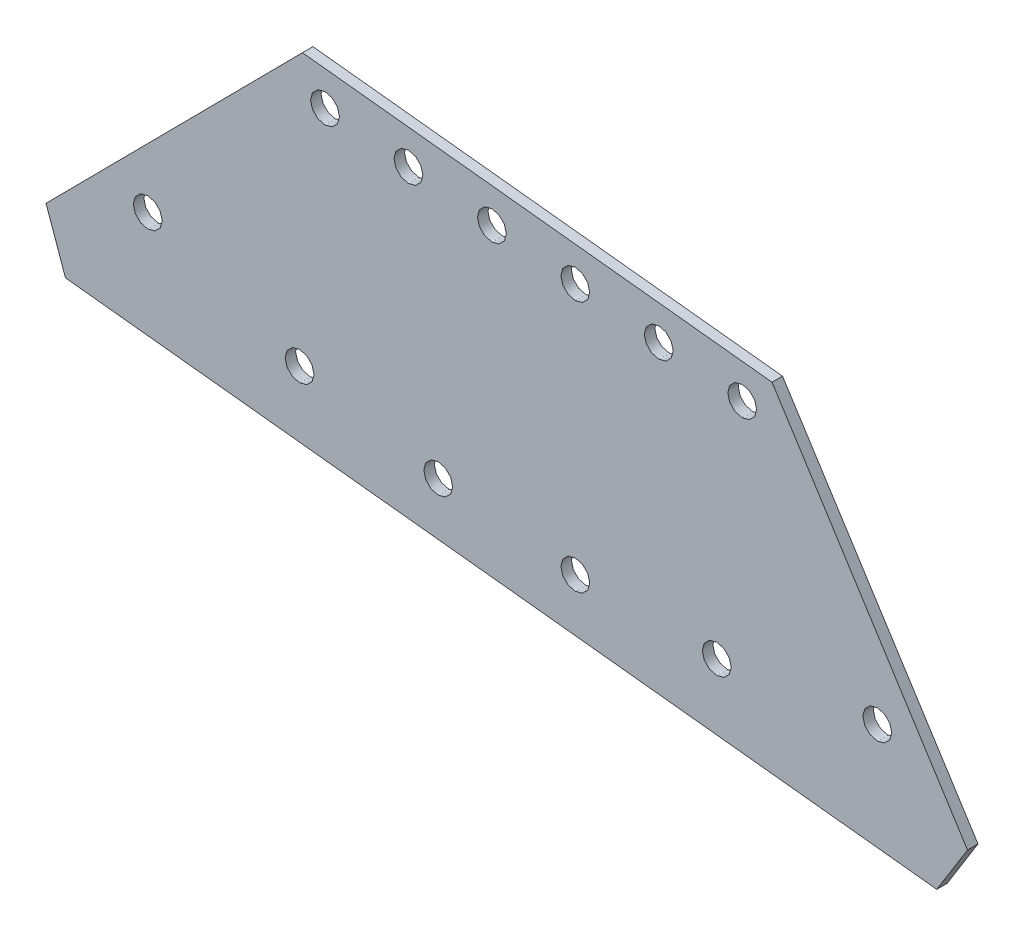
# Autodesk Inventor part: Endgame main polycarb
Saved by Autodesk Inventor 2023.2 (Build 272271030, 271C)
## iProperties
Created: 2023-04-06
Part Number: Endgame main polycarb
Material: Generic
Document SubType Name: Modeling
Designer: Main Account
Density: 1 g/cm^3
Appearance: Default
Author: Main Account
Autodesk Inventor part; units mm, degrees
ref_plane "YZ Plane" through (0, 0, 0) normal (1, 0, 0) x (0, 1, 0)
ref_plane "XZ Plane" through (0, 0, 0) normal (0, 1, 0) x (-1, 0, 0)
ref_plane "XY Plane" through (0, 0, 0) normal (0, 0, 1) x (1, 0, 0)
sketch "Sketch1" plane through (0, 0, 0) normal (0, 0, 1) x (1, 0, 0)
  circle A0 centre (31.6038, 86.1786) radius 2.1844 projected
  circle A1 centre (18.9769, 87.5393) radius 2.1844 projected
  circle A2 centre (6.35, 88.9) radius 2.1844 projected
  circle A3 centre (-6.2769, 90.2607) radius 2.1844 projected
  circle A4 centre (-18.9038, 91.6214) radius 2.1844 projected
  circle A5 centre (-31.5307, 92.9821) radius 2.1844 projected
  line L0 (36.1246, 90.903) -> (-34.9412, 98.5613)
  line L1 (-73.7518, 59.4167) -> (-34.9412, 98.5613)
  line L2 (36.1246, 90.903) -> (65.7044, 44.3885)
  line L3 (61.0548, 36.9038) -> (-70.8037, 51.1132)
  circle A6 centre (52.0487, 54.0287) radius 2.1844 projected
  circle A7 centre (27.7551, 50.4643) radius 2.1844 projected
  circle A8 centre (6.35, 50.8) radius 2.1844 projected
  circle A9 centre (-14.3942, 53.0355) radius 2.1844 projected
  circle A10 centre (-35.3794, 57.2679) radius 2.1844 projected
  circle A11 centre (-58.3558, 65.9262) radius 2.1844 projected
  line L4 (61.0548, 36.9038) -> (65.7044, 44.3885)
  line L5 (-70.8037, 51.1132) -> (-73.7518, 59.4167)
  point P0 (0, 0)
  point P1 (-80.9052, 52.2018)
  point P2 (71.1563, 35.8152)
  dimension "d2" = 10.16
  dimension "d3" = 10.16
  dimension "d4" = 10.16
  dimension "d5" = 10.16
  constraints: 12 end point, 4 point on line, 1 parallel, 4 other
  measures "d2" distance of L3.start point (71.156, 35.815)
  measures "d3" distance of L2.end point (71.156, 35.815)
  measures "d4" distance of L3.end point (-80.905, 52.202)
  measures "d5" distance of L1.start point (-80.905, 52.202)
extrude "Extrusion1" add sketch "Sketch1" along normal blind 1.5875
equation "\"d3\" = d2"
equation "\"d4\" = d2"
equation "\"d5\" = d4"
body "Solid1"
